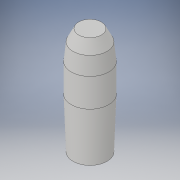
# Autodesk Inventor part: USBCamera
Saved by Autodesk Inventor 2019 (Build 230136000, 136)
## iProperties
Created: 2019-07-15
Part Number: USBCamera
Material: Generic
Document SubType Name: Modeling
Designer: aorfi
Density: 1 g/cm^3
Appearance: Default
Author: aorfi
Autodesk Inventor part; units mm, degrees
sketch "Sketch1" plane through (0, 0, 0) normal (0, 1, 0) x (-1, 0, 0)
  circle A0 centre (0, 0) radius 16.5
  dimension "d0" = 33
  constraints: 1 centre point, 1 coincident
  measures "d0" diameter of A0
extrude "Extrusion1" add sketch "Sketch1" along normal blind 25
ref_plane "Work Plane1" through (0, -44, 0) normal (0, -1, 0) x (1, 0, 0)
sketch "Sketch2" plane through (0, -44, 0) normal (0, -1, 0) x (1, 0, 0)
  circle A0 centre (0, 0) radius 15
  dimension "d4" = 30
  constraints: 1 centre point, 1 coincident
  measures "d4" diameter of A0
loft "Loft1" add profiles "Sketch2" section 1 edges at (16.5, 0, 0)
ref_plane "Work Plane2" through (0, 40, 0) normal (0, 1, 0) x (1, 0, 0)
sketch "Sketch3" plane through (0, 40, 0) normal (0, 1, 0) x (1, 0, 0)
  circle A0 centre (0, 0) radius 15
  dimension "d10" = 30
  constraints: 1 centre point, 1 coincident
  measures "d10" diameter of A0
loft "Loft2" add profiles "Sketch3" section 1 edges at (16.5, 25, 0)
ref_plane "Work Plane3" through (0, 50, 0) normal (0, 1, 0) x (1, 0, 0)
sketch "Sketch4" plane through (0, 50, 0) normal (0, 1, 0) x (1, 0, 0)
  circle A0 centre (0, 0) radius 10
  dimension "d16" = 20
  constraints: 1 centre point, 1 coincident
  measures "d16" diameter of A0
loft "Loft3" add profiles "Sketch4" section 1 edges at (15, 40, 0)
body "Solid1"
